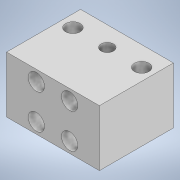
# Autodesk Inventor part: NewSinkV3
Saved by Autodesk Inventor 2020 (Build 240168000, 168)
## iProperties
Created: 2019-09-11
Part Number: NewSinkV3
Material: Generic
Document SubType Name: Modeling
Designer: colman
Density: 1 g/cm^3
Appearance: Default
Author: colman
Autodesk Inventor part; units mm, degrees
ref_plane "YZ Plane" through (0, 0, 0) normal (1, 0, 0) x (0, 1, 0)
ref_plane "XZ Plane" through (0, 0, 0) normal (0, 1, 0) x (-1, 0, 0)
ref_plane "XY Plane" through (0, 0, 0) normal (0, 0, 1) x (1, 0, 0)
sketch "Sketch1" plane through (0, 0, 0) normal (0, 0, 1) x (1, 0, 0)
  line L0 (8.25, 5) -> (-8.25, 5)
  line L1 (-8.25, 5) -> (-8.25, -5)
  line L2 (-8.25, -5) -> (8.25, -5)
  line L3 (8.25, -5) -> (8.25, 5)
  point P0 (0, 0)
  dimension "d19" = 10
  dimension "d36" = 16.5
  dimension "d37" = 5
  constraints: 8 end point, 2 parallel, 1 horizontal, 1 perpendicular
  measures "d19" distance of L1.end L0.end
  measures "d36" distance of L0.start L0.end
  measures "d37" distance from line of point (0, 0) L2
extrude "Box" add sketch "Sketch1" along normal blind 6.927 and the other way blind 6.223
sketch "Sketch3" plane through (0, 0, -6.223) normal (0, 0, -1) x (-1, 0, 0)
  line L0 (-5.08, 0) -> (5.08, 0) construction
  line L1 (-4.75, 0) -> (4.75, 0) construction
  circle A0 centre (0, 0) radius 2
  dimension "d35" = 4
  constraints: 8 end point, 2 midpoint, 2 point on line, 1 centre point, 1 coincident
  measures "d35" diameter of A0
extrude "Slot" cut sketch "Sketch3" against normal blind 11.15
sketch "Sketch4" plane through (0, 0, -6.223) normal (0, 0, -1) x (-1, 0, 0)
  circle A0 centre (-2.96, 3.0769) radius 1.45
  line L0 (8.25, 5) -> (-8.25, 5) projected
  circle A1 centre (0, 0) radius 2 projected
  line L1 (-8.25, 5) -> (-8.25, -5) projected
  dimension "d32" = 2.9
  dimension "d34" = 1.9231
  dimension "d39" = 5.29
  dimension "d40" = 5
  constraints: 1 centre point
  measures "d32" diameter of A0
  measures "d34" distance from line of A0.centre L0
  measures "d39" distance from line of L1 A0.centre
  measures "d40" distance from line of point (0, 0) L0
extrude "MountingHole" cut sketch "Sketch4" against normal blind 15 contours A0
pattern_linear "Mounting Holes" count 2 spacing 5.92 along (-1, 0, 0) count 2 spacing 6.154 along (0, -1, 0) of "MountingHole"
sketch "Sketch6" plane through (-8.25, 5, 6.927) normal (0, 1, 0) x (1, 0, 0)
  circle A0 centre (8.25, 9.65) radius 1.105
  line L0 (0, 13.15) -> (16.5, 13.15) projected
  dimension "d20" = 2.21
  dimension "d46" = 3.5
  constraints: 1 centre point
  measures "d20" diameter of A0
  measures "d46" distance from line of L0 A0.centre
extrude "CentralSMAHole" cut sketch "Sketch6" against normal blind 12
sketch "Sketch8" plane through (-8.25, 5, 6.927) normal (0, 1, 0) x (1, 0, 0)
  circle A0 centre (14.36, 9.65) radius 1.295
  line L0 (0, 13.15) -> (16.5, 13.15) projected
  dimension "d23" = 2.59
  dimension "d45" = 3.5
  constraints: 1 centre point
  measures "d23" diameter of A0
  measures "d45" distance from line of L0 A0.centre
extrude "SMAMounting" cut sketch "Sketch8" against normal blind 12
pattern_linear "SMAMountingHoles" count 2 spacing 12.22 along (-1, 0, 0) of "SMAMounting"
equation "\"d37\" = 0.5 * d19"
equation "\"d34\" = 0.384615 * d40"
body "Solid1"
